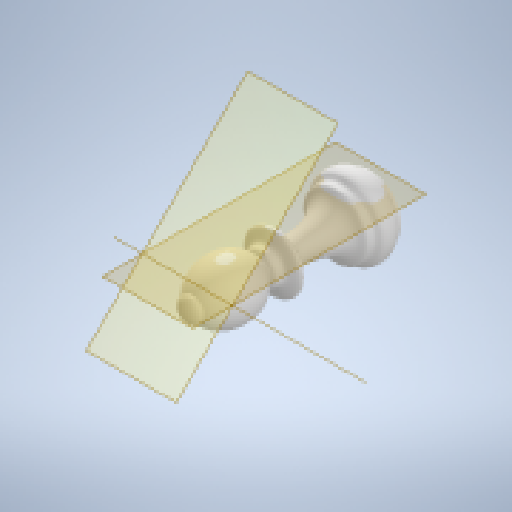
# Autodesk Inventor part: bishop-white
Saved by Autodesk Inventor 2024.1 (Build 281209000, 209)
## iProperties
Created: 2025-08-03
Part Number: bishop-white
Material: Generic
Document SubType Name: Modeling
Designer: iwheard
Density: 1 g/cm^3
Appearance: Default
Author: iwheard
Autodesk Inventor part; units mm, degrees
ref_plane "YZ Plane" through (0, 0, 0) normal (1, 0, 0) x (0, 1, 0)
ref_plane "XY Plane" through (0, 0, 0) normal (0, 0, 1) x (1, 0, 0)
sketch "Sketch1" plane through (0, 0, 0) normal (0, 0, 1) x (1, 0, 0)
  circle A0 centre (0, 25.5) radius 3
  circle A1 centre (0, 25.5) radius 5
  point P0 (0, 0)
  dimension "d0" = 10
  constraints: 2 centre point
  measures "d0" diameter of A1
extrude "Extrusion1" add sketch "Sketch1" along normal blind 3
sketch "Sketch3" plane through (0, 25.5, 3) normal (0, 0, 1) x (1, 0, 0)
  circle A0 centre (0, 0) radius 5 projected
  circle A1 centre (0, 0) radius 3 projected
  circle A2 centre (0, 0) radius 7.15
  point P0 (0, -25.5)
  dimension "d6" = 14.3
  constraints: 1 centre point
  measures "d6" diameter of A2
extrude "Extrusion2" add sketch "Sketch3" against normal blind 3 contours A2
sketch "Sketch2" plane through (0, 0, 0) normal (1, 0, 0) x (0, 1, 0)
  line L0 (30.5, 3) -> (20.5, 3) projected
  line L1 (30.5, 0) -> (20.5, 0) projected
  line L2 (30.5, 0) -> (30.5, 3) projected
  line L3 (28.5, 3) -> (28.5, 0) projected
  line L4 (32.65, 3) -> (18.35, 3) projected
  line L5 (32.65, 3) -> (32.65, 0) projected
  line L6 (28.3472, 21.8) -> (18.9472, 21.8)
  line L7 (19.95, 21.8) -> (32.25, 21.8)
  line L8 (32.65, 0.8) -> (33.5166, 1.2027) construction
  line L9 (33.5166, 1.2027) -> (34.0787, 2.2554) construction
  line L10 (34.0787, 2.2554) -> (34.4911, 4.0365) construction
  line L11 (34.4911, 4.0365) -> (34.2278, 5.2149) construction
  line L12 (34.2278, 5.2149) -> (33.7977, 5.9148) construction
  line L13 (33.7977, 5.9148) -> (33.0833, 6.0655) construction
  line L14 (33.0833, 6.0655) -> (32.65, 6.8872) construction
  line L15 (32.65, 6.8872) -> (33.4405, 8.43) construction
  line L16 (33.4405, 8.43) -> (29.4068, 8.43) construction
  line L17 (29.4068, 8.43) -> (27.9564, 17.9326) construction
  line L18 (32.25, 21.8) -> (32.25, 21.8) construction
  spline S0 degree 4 poles (32.65, 0.8) (33.5166, 1.2027) (34.0787, 2.2554) (34.4911, 4.0365) (34.2278, 5.2149) (33.7977, 5.9148) (33.0833, 6.0655) (32.65, 6.8872) (33.4405, 8.43) (29.4068, 8.43) (27.9564, 17.9326) (28.5, 20.0574) (31.3751, 21.1669) (32.1291, 21.5879) (32.2499, 21.7998) (32.25, 21.8) knots 1 1 1 1 1 2 3 4 5 6 7 8 9 10 10.505813 10.92418 11 11 11 11 11
  ellipse E0 centre (25.5, 41) end of major axis (22.7, 41) minor radius 1.4
  ellipse E1 centre (25.5, 33) end of major axis (25.5, 25) minor radius 6.5
  line L19 (32.25, 21.8) -> (32.4585, 22.7) construction
  line L20 (28.3607, 25.5724) -> (28.3108, 25.7867) construction
  spline S1 degree 4 poles (32.25, 21.8) (32.4585, 22.7) (29.8146, 23.2462) (29.2082, 23.4583) (29.4068, 25.3272) (28.3607, 25.5724) (28.3108, 25.7867) knots 1 1 1 1 1 1.620558 1.874487 2 2 2 2 2
  line L21 (29.4068, 25.3272) -> (28.3607, 25.5724) construction
  line L22 (32.4585, 22.7) -> (29.8146, 23.2462) construction
  line L23 (29.8146, 23.2462) -> (29.2082, 23.4583) construction
  line L24 (29.2082, 23.4583) -> (29.4068, 25.3272) construction
  line L25 (25.5, 42.4) -> (25.5, 3)
  line L26 (32.1291, 21.5879) -> (32.25, 21.8) construction
  line L27 (27.9564, 17.9326) -> (28.5, 20.0574) construction
  line L28 (28.5, 20.0574) -> (31.3751, 21.1669) construction
  line L29 (31.3751, 21.1669) -> (32.1291, 21.5879) construction
  point P0 (0, 0)
  point P1 (25.5, 0)
  point P2 (25.5, 3)
  point P3 (28.01, 40.3795)
  dimension "d127" = 2.8
  dimension "d128" = 1.4
  dimension "d129" = 6.5
  dimension "d130" = 8
  dimension "d89" = 12.3
  dimension "d131" = 8
  dimension "d132" = 33
  dimension "d133" = 11.2
  dimension "d134" = 6.75
  dimension "d135" = 0.8
  constraints: 6 end point, 3 midpoint, 3 vertical alignment, 2 coincident, 1 horizontal, 1 horizontal alignment, 1 point on line, 14 other
  measures "d89" distance of L7.end L7.start
  measures "d131" distance of point (25.5, 33) point (25.5, 41)
  measures "d132" distance from line of L1 point (25.5, 33)
  measures "d133" distance from line of point (25.5, 33) L6
  measures "d134" horizontal distance of point (32.25, 21.8) point (25.5, 33)
  measures "d135" distance from line of L8.start L1
revolve "Revolution1" add sketch "Sketch2" angle 360 about axis through (0, 25.5, 42.4) along (0, 0, -1) picked at (27.4668, 31.4146) picked at (26.1235, 40.0751) picked at (25.9921, 41.4318) contours L0 L25 L6 L7 S0 L5 L4 | L25 E1 S1 L7 L6 | L25 E0 E1 | L25 E1 E0 | E1 L25 E0
fillet "Fillet5" radius 0.6 1 edges at (0, 18.75, 21.8)
ref_plane "Work Plane6" through (0, 32, 33) normal (0, 1, 0) x (-1, 0, 0)
ref_plane "Work Plane9" through (0, 49.6777, 17.6777) normal (0, 0.7071068, 0.7071068) x (1, 0, 0)
ref_plane "Work Plane7" through (0, 32, 0) normal (0, 0.7071068, 0.7071068) x (1, 0, 0)
sketch "Sketch16" plane through (0, 49.6777, 17.6777) normal (0, 0.7071068, 0.7071068) x (1, 0, 0)
  line L0 (8, -30.0355) -> (0, -26.3614) construction
  line L1 (0, -26.3614) -> (-8, -30.0129) construction
  spline S0 degree 2 poles (8, -30.0355) (0, -26.3614) (-8, -30.0129) knots 1 1 1 2 2 2
  line L2 (8, -30.0355) -> (7.5, -28.6475)
  line L3 (-7.5, -28.6274) -> (-8, -30.0129)
  spline S1 degree 5 poles (7.5, -28.6475) (6.0737, -28.0663) (4.5989, -27.6042) (3.0818, -27.2819) (0.0019, -26.958) (-3.0789, -27.2731) (-4.5967, -27.5912) (-6.0725, -28.0496) (-7.5, -28.6274) knots 0 0 0 0 0 0 0.500029 0.500029 0.500029 1 1 1 1 1 1
  point P0 (0, -22.6274)
  point P1 (7.6736, -28.7905)
  point P2 (-7.681, -28.8125)
  point P3 (-4, -29.7611)
  point P4 (4, -29.7611)
  dimension "d137" = 8
  dimension "d138" = 8
  dimension "d141" = 6
  dimension "d142" = 7.5
  dimension "d143" = 7.5
  constraints: 4 end point, 1 vertical alignment, 6 other
  measures "d137" horizontal distance of L1.end point (0, -22.627)
  measures "d138" horizontal distance of L0.start point (0, -22.627)
  measures "d141" vertical distance of point (0, -22.627) L3.start
  measures "d142" horizontal distance of point (0, -22.627) L2.end
  measures "d143" horizontal distance of point (0, -22.627) L3.start
sketch "Sketch17" plane through (0, 0, 0) normal (1, 0, 0) x (0, 1, 0)
  line L0 (29.024, 39.7222) -> (29.1615, 34.9225) construction
  line L1 (29.1615, 34.9225) -> (26.7953, 31.6689) construction
  spline S0 degree 2 poles (29.024, 39.7222) (29.1615, 34.9225) (26.7953, 31.6689) knots 1 1 1 2 2 2
  point P0 (0, 0)
  constraints: 3 other
sweep "Sweep1" cut profiles "Sketch16" path "Sketch17"
sketch "Sketch15" plane through (0, 31.8, 41.7) normal (0, 0.7071068, -0.7071068) x (-1, 0, 0)
  line L0 (0, 3.0363) -> (2.0785, -0.5637)
  line L1 (2.0785, -0.5637) -> (-2.0785, -0.5637)
  line L2 (-2.0785, -0.5637) -> (0, 3.0363)
  ellipse E0 centre (0, -4.4548) end of major axis (-4.0302, -4.4548) minor radius 2.8498 projected
  ellipse E1 centre (0, -4.4548) end of major axis (-6.3, -4.4548) minor radius 4.4548 projected
  line L3 (2.0785, -0.5637) -> (0, -4.1637)
  line L4 (0, -4.1637) -> (-2.0785, -0.5637)
  line L5 (-2.0785, -0.5637) -> (2.0785, -0.5637)
  point P0 (0, -51.9723)
  point P1 (0, -14.238)
  point P2 (0, 0.6363)
  point P3 (0, -10.0471)
  point P4 (0, -1.7637)
  dimension "d118" = 2.4
  dimension "d51" = 6.0425
  dimension "d52" = 2.3149
  dimension "d53" = 2.4891
  dimension "d54" = 7.8751
  dimension "d55" = 5.9159
  dimension "d57" = 0.4873
  dimension "d58" = 0.2598
  dimension "d59" = 1.3529
  dimension "d60" = 2.0044
  dimension "d61" = 0.4355
  constraints: 72 end point, 18 parallel, 9 perpendicular, 6 point on line, 1 midpoint
sketch "Sketch12" plane through (-2.1873, 31.7347, 5.7495) normal (0, 0.6767574, 0.7362061) x (1, 0, 0)
  line L0 (7.0778, 4.6058) -> (7.2853, 4.1237)
  line L1 (7.2853, 4.1237) -> (7.7383, 3.6103)
  line L2 (7.7383, 3.6103) -> (8.2511, 3.1473)
  line L3 (8.2511, 3.1473) -> (8.8771, 3.0178)
  line L4 (8.8771, 3.0178) -> (9.2618, 2.9917)
  line L5 (9.2618, 2.9917) -> (9.5367, 3.0866)
  line L6 (9.5367, 3.0866) -> (10.2847, 4.0131)
  line L7 (10.2847, 4.0131) -> (10.6933, 4.6314)
  line L8 (10.6933, 4.6314) -> (10.7522, 4.8215)
  line L9 (10.7522, 4.8215) -> (10.6935, 4.9491)
  line L10 (10.6935, 4.9491) -> (10.1629, 5.066)
  line L11 (10.1629, 5.066) -> (8.9792, 5.0827)
  line L12 (8.9792, 5.0827) -> (7.1904, 5.0231)
  line L13 (7.1904, 5.0231) -> (7.0137, 4.8815)
  line L14 (7.0137, 4.8815) -> (7.0778, 4.6058)
  line L15 (-7.9123, 3.5374) -> (-6.7126, 2.2089)
  line L16 (-6.7126, 2.2089) -> (-6.4779, 2.096)
  line L17 (-6.4779, 2.096) -> (-6.283, 2.1812)
  line L18 (-6.283, 2.1812) -> (-5.9921, 2.5161)
  line L19 (-5.9921, 2.5161) -> (-5.7627, 3.7265)
  line L20 (-5.7627, 3.7265) -> (-5.6649, 4.5105)
  line L21 (-5.6649, 4.5105) -> (-5.802, 4.9132)
  line L22 (-5.802, 4.9132) -> (-6.3268, 5.0615)
  line L23 (-6.3268, 5.0615) -> (-7.392, 5.0827)
  line L24 (-7.392, 5.0827) -> (-8.4398, 5.0585)
  line L25 (-8.4398, 5.0585) -> (-8.8433, 4.8895)
  line L26 (-8.8433, 4.8895) -> (-8.6512, 4.4308)
  line L27 (-8.6512, 4.4308) -> (-7.9123, 3.5374)
  line L28 (0.8872, 3.9133) -> (0.9729, 2.8417)
  line L29 (0.9729, 2.8417) -> (1.3707, 2.3566)
  line L30 (1.3707, 2.3566) -> (1.8274, 2.0403)
  line L31 (1.8274, 2.0403) -> (2.3257, 2.1498)
  line L32 (2.3257, 2.1498) -> (2.6211, 2.2757)
  line L33 (2.6211, 2.2757) -> (2.7942, 2.4798)
  line L34 (2.7942, 2.4798) -> (3.0423, 3.7065)
  line L35 (3.0423, 3.7065) -> (3.1457, 4.5021)
  line L36 (3.1457, 4.5021) -> (3.0772, 4.9107)
  line L37 (3.0772, 4.9107) -> (2.7441, 5.0612)
  line L38 (2.7441, 5.0612) -> (2.0536, 5.0827)
  line L39 (2.0536, 5.0827) -> (1.3603, 5.0644)
  line L40 (1.3603, 5.0644) -> (1.0077, 4.9365)
  line L41 (1.0077, 4.9365) -> (0.8864, 4.5894)
  line L42 (0.8864, 4.5894) -> (0.8872, 3.9133)
  line L43 (-2.0027, 3.87) -> (-1.9541, 3.154)
  line L44 (-1.9541, 3.154) -> (-1.7644, 2.7594)
  line L45 (-1.7644, 2.7594) -> (-1.3586, 2.5882)
  line L46 (-1.3586, 2.5882) -> (-0.6615, 2.5421)
  line L47 (-0.6615, 2.5421) -> (0.3743, 2.5372)
  line L48 (0.3743, 2.5372) -> (0.6823, 2.6332)
  line L49 (0.6823, 2.6332) -> (0.8414, 2.878)
  line L50 (0.8414, 2.878) -> (0.8353, 3.9144)
  line L51 (0.8353, 3.9144) -> (0.7939, 4.5898)
  line L52 (0.7939, 4.5898) -> (0.6303, 4.9367)
  line L53 (0.6303, 4.9367) -> (0.2097, 5.0644)
  line L54 (0.2097, 5.0644) -> (-0.6026, 5.0827)
  line L55 (-0.6026, 5.0827) -> (-1.4144, 5.0637)
  line L56 (-1.4144, 5.0637) -> (-1.8308, 4.9311)
  line L57 (-1.8308, 4.9311) -> (-1.9832, 4.5711)
  line L58 (-1.9832, 4.5711) -> (-2.0027, 3.87)
  line L59 (-4.1807, 3.6112) -> (-4.1404, 2.7644)
  line L60 (-4.1404, 2.7644) -> (-4.0148, 2.3547)
  line L61 (-4.0148, 2.3547) -> (-3.7027, 2.2674)
  line L62 (-3.7027, 2.2674) -> (-3.1032, 2.3879)
  line L63 (-3.1032, 2.3879) -> (-2.4946, 2.5599)
  line L64 (-2.4946, 2.5599) -> (-2.1825, 2.7714)
  line L65 (-2.1825, 2.7714) -> (-2.0686, 3.161)
  line L66 (-2.0686, 3.161) -> (-2.0545, 3.8676)
  line L67 (-2.0545, 3.8676) -> (-2.0739, 4.5701)
  line L68 (-2.0739, 4.5701) -> (-2.1934, 4.9308)
  line L69 (-2.1934, 4.9308) -> (-2.515, 5.0637)
  line L70 (-2.515, 5.0637) -> (-3.1405, 5.0827)
  line L71 (-3.1405, 5.0827) -> (-3.7652, 5.0597)
  line L72 (-3.7652, 5.0597) -> (-4.0818, 4.8988)
  line L73 (-4.0818, 4.8988) -> (-4.1878, 4.4619)
  line L74 (-4.1878, 4.4619) -> (-4.1807, 3.6112)
  line L75 (-5.1318, 2.1686) -> (-4.4254, 1.9987)
  line L76 (-4.4254, 1.9987) -> (-4.2625, 2.0403)
  line L77 (-4.2625, 2.0403) -> (-4.2322, 3.5999)
  line L78 (-4.2322, 3.5999) -> (-4.3449, 4.8973)
  line L79 (-4.3449, 4.8973) -> (-4.5302, 5.0595)
  line L80 (-4.5302, 5.0595) -> (-4.8826, 5.0827)
  line L81 (-4.8826, 5.0827) -> (-5.2378, 5.0615)
  line L82 (-5.2378, 5.0615) -> (-5.4424, 4.9134)
  line L83 (-5.4424, 4.9134) -> (-5.7099, 3.7282)
  line L84 (-5.7099, 3.7282) -> (-5.824, 2.9419)
  line L85 (-5.824, 2.9419) -> (-5.8018, 2.5174)
  line L86 (-5.8018, 2.5174) -> (-5.5891, 2.3084)
  line L87 (-5.5891, 2.3084) -> (-5.1318, 2.1686)
  line L88 (3.6495, 2.0407) -> (4.1162, 1.9046)
  line L89 (4.1162, 1.9046) -> (4.4149, 2.0092)
  line L90 (4.4149, 2.0092) -> (4.6182, 2.4772)
  line L91 (4.6182, 2.4772) -> (4.7988, 3.4316)
  line L92 (4.7988, 3.4316) -> (4.9342, 4.3861)
  line L93 (4.9342, 4.3861) -> (4.915, 4.8762)
  line L94 (4.915, 4.8762) -> (4.6833, 5.0568)
  line L95 (4.6833, 5.0568) -> (4.1814, 5.0827)
  line L96 (4.1814, 5.0827) -> (3.6721, 5.0612)
  line L97 (3.6721, 5.0612) -> (3.3891, 4.9105)
  line L98 (3.3891, 4.9105) -> (3.2305, 4.5016)
  line L99 (3.2305, 4.5016) -> (3.0945, 3.7053)
  line L100 (3.0945, 3.7053) -> (2.9842, 2.9046)
  line L101 (2.9842, 2.9046) -> (3.0052, 2.4643)
  line L102 (3.0052, 2.4643) -> (3.2097, 2.2283)
  line L103 (3.2097, 2.2283) -> (3.6495, 2.0407)
  line L104 (9.8736, 2.3824) -> (10.0725, 2.0726)
  line L105 (10.0725, 2.0726) -> (10.3077, 1.9004)
  line L106 (10.3077, 1.9004) -> (11.4946, 1.7208)
  line L107 (11.4946, 1.7208) -> (12.2533, 1.6733)
  line L108 (12.2533, 1.6733) -> (12.6429, 1.8259)
  line L109 (12.6429, 1.8259) -> (12.7865, 2.33)
  line L110 (12.7865, 2.33) -> (12.8069, 3.3371)
  line L111 (12.8069, 3.3371) -> (12.7937, 4.3463)
  line L112 (12.7937, 4.3463) -> (12.701, 4.8645)
  line L113 (12.701, 4.8645) -> (12.4492, 5.0554)
  line L114 (12.4492, 5.0554) -> (11.959, 5.0827)
  line L115 (11.959, 5.0827) -> (11.4567, 5.0658)
  line L116 (11.4567, 5.0658) -> (11.1204, 4.9472)
  line L117 (11.1204, 4.9472) -> (10.338, 3.9987)
  line L118 (10.338, 3.9987) -> (9.7002, 2.9837)
  line L119 (9.7002, 2.9837) -> (9.7073, 2.7071)
  line L120 (9.7073, 2.7071) -> (9.8736, 2.3824)
  line L121 (4.9302, 1.5607) -> (5.2883, 1.3935)
  line L122 (5.2883, 1.3935) -> (5.7656, 1.4894)
  line L123 (5.7656, 1.4894) -> (6.0603, 1.5897)
  line L124 (6.0603, 1.5897) -> (6.2588, 1.7671)
  line L125 (6.2588, 1.7671) -> (6.7286, 2.8722)
  line L126 (6.7286, 2.8722) -> (7.1151, 4.0203)
  line L127 (7.1151, 4.0203) -> (7.0251, 4.5992)
  line L128 (7.0251, 4.5992) -> (6.768, 5.0224)
  line L129 (6.768, 5.0224) -> (5.9825, 5.0828)
  line L130 (5.9825, 5.0828) -> (5.4735, 5.0569)
  line L131 (5.4735, 5.0569) -> (5.1859, 4.8758)
  line L132 (5.1859, 4.8758) -> (5.0136, 4.3843)
  line L133 (5.0136, 4.3843) -> (4.8506, 3.4272)
  line L134 (4.8506, 3.4272) -> (4.6667, 1.9523)
  line L135 (4.6667, 1.9523) -> (4.7388, 1.7086)
  line L136 (4.7388, 1.7086) -> (4.9302, 1.5607)
  line L137 (-10.0996, 2.0946) -> (-9.1658, 1.7122)
  line L138 (-9.1658, 1.7122) -> (-7.9691, 1.6823)
  line L139 (-7.9691, 1.6823) -> (-6.8767, 1.7227)
  line L140 (-6.8767, 1.7227) -> (-6.6741, 1.8325)
  line L141 (-6.6741, 1.8325) -> (-6.7946, 2.1343)
  line L142 (-6.7946, 2.1343) -> (-7.9643, 3.5183)
  line L143 (-7.9643, 3.5183) -> (-9.2457, 4.8871)
  line L144 (-9.2457, 4.8871) -> (-9.6422, 5.0582)
  line L145 (-9.6422, 5.0582) -> (-10.1491, 5.0827)
  line L146 (-10.1491, 5.0827) -> (-10.6349, 5.0628)
  line L147 (-10.6349, 5.0628) -> (-10.8844, 4.9235)
  line L148 (-10.8844, 4.9235) -> (-10.9763, 4.5454)
  line L149 (-10.9763, 4.5454) -> (-10.9894, 3.8092)
  line L150 (-10.9894, 3.8092) -> (-10.9755, 3.0661)
  line L151 (-10.9755, 3.0661) -> (-10.8782, 2.6398)
  line L152 (-10.8782, 2.6398) -> (-10.614, 2.3696)
  line L153 (-10.614, 2.3696) -> (-10.0996, 2.0946)
  line L154 (7.0017, 1.241) -> (7.63, 0.9268)
  line L155 (7.63, 0.9268) -> (7.9057, 0.9992)
  line L156 (7.9057, 0.9992) -> (8.0999, 1.239)
  line L157 (8.0999, 1.239) -> (8.1581, 2.0966)
  line L158 (8.1581, 2.0966) -> (8.1291, 3.0002)
  line L159 (8.1291, 3.0002) -> (7.7126, 3.5622)
  line L160 (7.7126, 3.5622) -> (7.4273, 3.835)
  line L161 (7.4273, 3.835) -> (7.2344, 3.8511)
  line L162 (7.2344, 3.8511) -> (6.7731, 2.8435)
  line L163 (6.7731, 2.8435) -> (6.5187, 2.1301)
  line L164 (6.5187, 2.1301) -> (6.4577, 1.7254)
  line L165 (6.4577, 1.7254) -> (6.6116, 1.4791)
  line L166 (6.6116, 1.4791) -> (7.0017, 1.241)
  line L167 (8.7073, 1.062) -> (9.229, 1.0437)
  line L168 (9.229, 1.0437) -> (9.6868, 1.4053)
  line L169 (9.6868, 1.4053) -> (10.0394, 1.8435)
  line L170 (10.0394, 1.8435) -> (9.8261, 2.3611)
  line L171 (9.8261, 2.3611) -> (9.4772, 2.8348)
  line L172 (9.4772, 2.8348) -> (8.8815, 2.9651)
  line L173 (8.8815, 2.9651) -> (8.5129, 2.9925)
  line L174 (8.5129, 2.9925) -> (8.32, 2.9106)
  line L175 (8.32, 2.9106) -> (8.2098, 2.0909)
  line L176 (8.2098, 2.0909) -> (8.2457, 1.2518)
  line L177 (8.2457, 1.2518) -> (8.4, 1.124)
  line L178 (8.4, 1.124) -> (8.7073, 1.062)
  line L179 (-1.1975, 1.7234) -> (-0.675, 1.0352)
  line L180 (-0.675, 1.0352) -> (-0.4723, 0.9445)
  line L181 (-0.4723, 0.9445) -> (-0.2927, 1.0469)
  line L182 (-0.2927, 1.0469) -> (0.0688, 1.7112)
  line L183 (0.0688, 1.7112) -> (0.2778, 2.1497)
  line L184 (0.2778, 2.1497) -> (0.2719, 2.377)
  line L185 (0.2719, 2.377) -> (-0.0168, 2.4662)
  line L186 (-0.0168, 2.4662) -> (-0.6564, 2.4901)
  line L187 (-0.6564, 2.4901) -> (-1.2932, 2.4899)
  line L188 (-1.2932, 2.4899) -> (-1.5618, 2.41)
  line L189 (-1.5618, 2.41) -> (-1.513, 2.1784)
  line L190 (-1.513, 2.1784) -> (-1.1975, 1.7234)
  line L191 (-4.195, 1.1684) -> (-4.1205, 0.7334)
  line L192 (-4.1205, 0.7334) -> (-3.9979, 0.5322)
  line L193 (-3.9979, 0.5322) -> (-3.7448, 0.5165)
  line L194 (-3.7448, 0.5165) -> (-3.2787, 0.6377)
  line L195 (-3.2787, 0.6377) -> (-2.5542, 0.947)
  line L196 (-2.5542, 0.947) -> (-2.2838, 1.7234)
  line L197 (-2.2838, 1.7234) -> (-2.1873, 2.2134)
  line L198 (-2.1873, 2.2134) -> (-2.2423, 2.44)
  line L199 (-2.2423, 2.44) -> (-2.5269, 2.4601)
  line L200 (-2.5269, 2.4601) -> (-3.1198, 2.3307)
  line L201 (-3.1198, 2.3307) -> (-4.2248, 2.0047)
  line L202 (-4.2248, 2.0047) -> (-4.195, 1.1684)
  line L203 (0.319, 0.4663) -> (0.6686, 0.2086)
  line L204 (0.6686, 0.2086) -> (0.8924, 0.1637)
  line L205 (0.8924, 0.1637) -> (1.087, 0.3684)
  line L206 (1.087, 0.3684) -> (1.3488, 0.8597)
  line L207 (1.3488, 0.8597) -> (1.6779, 1.8428)
  line L208 (1.6779, 1.8428) -> (1.593, 2.0742)
  line L209 (1.593, 2.0742) -> (1.3408, 2.314)
  line L210 (1.3408, 2.314) -> (0.9255, 2.6376)
  line L211 (0.9255, 2.6376) -> (0.7075, 2.5879)
  line L212 (0.7075, 2.5879) -> (0.4957, 2.3936)
  line L213 (0.4957, 2.3936) -> (0.1242, 1.7056)
  line L214 (0.1242, 1.7056) -> (-0.15, 0.973)
  line L215 (-0.15, 0.973) -> (-0.0175, 0.7495)
  line L216 (-0.0175, 0.7495) -> (0.319, 0.4663)
  line L217 (2.5187, 0.9763) -> (2.9216, 0.5547)
  line L218 (2.9216, 0.5547) -> (3.1879, 0.4137)
  line L219 (3.1879, 0.4137) -> (3.4364, 0.5525)
  line L220 (3.4364, 0.5525) -> (3.7858, 0.9708)
  line L221 (3.7858, 0.9708) -> (4.1127, 1.4052)
  line L222 (4.1127, 1.4052) -> (4.2037, 1.6573)
  line L223 (4.2037, 1.6573) -> (4.0425, 1.823)
  line L224 (4.0425, 1.823) -> (3.6129, 1.9991)
  line L225 (3.6129, 1.9991) -> (2.8855, 2.2254)
  line L226 (2.8855, 2.2254) -> (2.3473, 2.1025)
  line L227 (2.3473, 2.1025) -> (2.0633, 1.8728)
  line L228 (2.0633, 1.8728) -> (1.9865, 1.679)
  line L229 (1.9865, 1.679) -> (2.5187, 0.9763)
  line L230 (-6.6273, 0.9505) -> (-6.5332, 0.2753)
  line L231 (-6.5332, 0.2753) -> (-6.2216, -0.0684)
  line L232 (-6.2216, -0.0684) -> (-5.6991, -0.3658)
  line L233 (-5.6991, -0.3658) -> (-4.8336, 0.0157)
  line L234 (-4.8336, 0.0157) -> (-4.242, 0.4515)
  line L235 (-4.242, 0.4515) -> (-4.2462, 1.1599)
  line L236 (-4.2462, 1.1599) -> (-4.437, 1.8453)
  line L237 (-4.437, 1.8453) -> (-5.1517, 2.1202)
  line L238 (-5.1517, 2.1202) -> (-5.8919, 2.2767)
  line L239 (-5.8919, 2.2767) -> (-6.2614, 2.1336)
  line L240 (-6.2614, 2.1336) -> (-6.627, 1.8108)
  line L241 (-6.627, 1.8108) -> (-6.6273, 0.9505)
  line L242 (-6.6273, 0.9505) -> (-6.6273, 0.9505)
  line L243 (-1.9958, 0.4442) -> (-1.5615, 0.1379)
  line L244 (-1.5615, 0.1379) -> (-1.1159, 0.4715)
  line L245 (-1.1159, 0.4715) -> (-0.8663, 0.7386)
  line L246 (-0.8663, 0.7386) -> (-0.7977, 0.9571)
  line L247 (-0.7977, 0.9571) -> (-1.2554, 1.7148)
  line L248 (-1.2554, 1.7148) -> (-1.7069, 2.2125)
  line L249 (-1.7069, 2.2125) -> (-1.9588, 2.3798)
  line L250 (-1.9588, 2.3798) -> (-2.1026, 2.2179)
  line L251 (-2.1026, 2.2179) -> (-2.2295, 1.7281)
  line L252 (-2.2295, 1.7281) -> (-2.3493, 0.9143)
  line L253 (-2.3493, 0.9143) -> (-1.9958, 0.4442)
  line L254 (-8.5605, 0.7102) -> (-7.9464, -0.0451)
  line L255 (-7.9464, -0.0451) -> (-7.6823, -0.0821)
  line L256 (-7.6823, -0.0821) -> (-7.2878, 0.0218)
  line L257 (-7.2878, 0.0218) -> (-6.7123, 0.2899)
  line L258 (-6.7123, 0.2899) -> (-6.6787, 0.9424)
  line L259 (-6.6787, 0.9424) -> (-6.7305, 1.3563)
  line L260 (-6.7305, 1.3563) -> (-6.8803, 1.566)
  line L261 (-6.8803, 1.566) -> (-7.9513, 1.6308)
  line L262 (-7.9513, 1.6308) -> (-8.6448, 1.6006)
  line L263 (-8.6448, 1.6006) -> (-8.9394, 1.4946)
  line L264 (-8.9394, 1.4946) -> (-8.8923, 1.2266)
  line L265 (-8.8923, 1.2266) -> (-8.5605, 0.7102)
  line L266 (9.5166, 0.3752) -> (9.6778, 0.049)
  line L267 (9.6778, 0.049) -> (9.9152, -0.0926)
  line L268 (9.9152, -0.0926) -> (11.2805, 0.0602)
  line L269 (11.2805, 0.0602) -> (12.6162, 0.3608)
  line L270 (12.6162, 0.3608) -> (12.7831, 0.5703)
  line L271 (12.7831, 0.5703) -> (12.807, 0.9279)
  line L272 (12.807, 0.9279) -> (12.7864, 1.2835)
  line L273 (12.7864, 1.2835) -> (12.6425, 1.4792)
  line L274 (12.6425, 1.4792) -> (11.4914, 1.669)
  line L275 (11.4914, 1.669) -> (10.2842, 1.7291)
  line L276 (10.2842, 1.7291) -> (10.0072, 1.6167)
  line L277 (10.0072, 1.6167) -> (9.7274, 1.3724)
  line L278 (9.7274, 1.3724) -> (9.3649, 0.9281)
  line L279 (9.3649, 0.9281) -> (9.5166, 0.3752)
  line L280 (1.3913, -0.4022) -> (1.8487, -0.6499)
  line L281 (1.8487, -0.6499) -> (2.4597, -0.593)
  line L282 (2.4597, -0.593) -> (3.0216, -0.4573)
  line L283 (3.0216, -0.4573) -> (3.1352, -0.1535)
  line L284 (3.1352, -0.1535) -> (3.0845, 0.23)
  line L285 (3.0845, 0.23) -> (2.4959, 0.9243)
  line L286 (2.4959, 0.9243) -> (2.097, 1.3422)
  line L287 (2.097, 1.3422) -> (1.8481, 1.4698)
  line L288 (1.8481, 1.4698) -> (1.6448, 1.2966)
  line L289 (1.6448, 1.2966) -> (1.3828, 0.812)
  line L290 (1.3828, 0.812) -> (1.0664, -0.0265)
  line L291 (1.0664, -0.0265) -> (1.1483, -0.2153)
  line L292 (1.1483, -0.2153) -> (1.3913, -0.4022)
  line L293 (5.3624, 0.5254) -> (5.5243, -0.1888)
  line L294 (5.5243, -0.1888) -> (6.2364, -0.5262)
  line L295 (6.2364, -0.5262) -> (6.9598, -0.7576)
  line L296 (6.9598, -0.7576) -> (7.2022, -0.7304)
  line L297 (7.2022, -0.7304) -> (7.3626, -0.5765)
  line L298 (7.3626, -0.5765) -> (7.5125, 0.0792)
  line L299 (7.5125, 0.0792) -> (7.5557, 0.7738)
  line L300 (7.5557, 0.7738) -> (6.9699, 1.1993)
  line L301 (6.9699, 1.1993) -> (6.3038, 1.5151)
  line L302 (6.3038, 1.5151) -> (5.7857, 1.4412)
  line L303 (5.7857, 1.4412) -> (5.3626, 1.2226)
  line L304 (5.3626, 1.2226) -> (5.3624, 0.5254)
  line L305 (3.2595, -0.5938) -> (4.0875, -0.7338)
  line L306 (4.0875, -0.7338) -> (4.7497, -0.7393)
  line L307 (4.7497, -0.7393) -> (5.0922, -0.5185)
  line L308 (5.0922, -0.5185) -> (5.3364, -0.1945)
  line L309 (5.3364, -0.1945) -> (5.3106, 0.5231)
  line L310 (5.3106, 0.5231) -> (5.206, 1.235)
  line L311 (5.206, 1.235) -> (4.8994, 1.5188)
  line L312 (4.8994, 1.5188) -> (4.6179, 1.6134)
  line L313 (4.6179, 1.6134) -> (4.4124, 1.5846)
  line L314 (4.4124, 1.5846) -> (3.8274, 0.9398)
  line L315 (3.8274, 0.9398) -> (3.2964, 0.23)
  line L316 (3.2964, 0.23) -> (3.1867, -0.1601)
  line L317 (3.1867, -0.1601) -> (3.1662, -0.467)
  line L318 (3.1662, -0.467) -> (3.2595, -0.5938)
  line L319 (-9.8289, -0.9114) -> (-8.7715, -0.9751)
  line L320 (-8.7715, -0.9751) -> (-8.5448, -0.866)
  line L321 (-8.5448, -0.866) -> (-8.3325, -0.6274)
  line L322 (-8.3325, -0.6274) -> (-8.148, -0.3726)
  line L323 (-8.148, -0.3726) -> (-8.1159, -0.1496)
  line L324 (-8.1159, -0.1496) -> (-8.6149, 0.698)
  line L325 (-8.6149, 0.698) -> (-9.2656, 1.548)
  line L326 (-9.2656, 1.548) -> (-10.1113, 2.0426)
  line L327 (-10.1113, 2.0426) -> (-10.6189, 2.2688)
  line L328 (-10.6189, 2.2688) -> (-10.8797, 2.2199)
  line L329 (-10.8797, 2.2199) -> (-10.9757, 1.7841)
  line L330 (-10.9757, 1.7841) -> (-10.9894, 0.8493)
  line L331 (-10.9894, 0.8493) -> (-10.9713, -0.0942)
  line L332 (-10.9713, -0.0942) -> (-10.8444, -0.5922)
  line L333 (-10.8444, -0.5922) -> (-10.4998, -0.8096)
  line L334 (-10.4998, -0.8096) -> (-9.8289, -0.9114)
  line L335 (8.2447, -1.1136) -> (8.7357, -1.3578)
  line L336 (8.7357, -1.3578) -> (9.0302, -1.4084)
  line L337 (9.0302, -1.4084) -> (9.2246, -1.2525)
  line L338 (9.2246, -1.2525) -> (9.4153, -0.8771)
  line L339 (9.4153, -0.8771) -> (9.643, -0.234)
  line L340 (9.643, -0.234) -> (9.4699, 0.3524)
  line L341 (9.4699, 0.3524) -> (9.1927, 0.8676)
  line L342 (9.1927, 0.8676) -> (8.6918, 1.0119)
  line L343 (8.6918, 1.0119) -> (8.1934, 1.0667)
  line L344 (8.1934, 1.0667) -> (7.9333, 0.9553)
  line L345 (7.9333, 0.9553) -> (7.7219, 0.7411)
  line L346 (7.7219, 0.7411) -> (7.5646, 0.0757)
  line L347 (7.5646, 0.0757) -> (7.4918, -0.3594)
  line L348 (7.4918, -0.3594) -> (7.5384, -0.6284)
  line L349 (7.5384, -0.6284) -> (8.2447, -1.1136)
  line L350 (-3.269, -0.6766) -> (-2.5401, -1.5703)
  line L351 (-2.5401, -1.5703) -> (-2.3211, -1.6435)
  line L352 (-2.3211, -1.6435) -> (-2.046, -1.5805)
  line L353 (-2.046, -1.5805) -> (-1.6478, -1.3713)
  line L354 (-1.6478, -1.3713) -> (-1.5901, -0.7296)
  line L355 (-1.5901, -0.7296) -> (-1.6439, -0.0529)
  line L356 (-1.6439, -0.0529) -> (-2.0264, 0.4018)
  line L357 (-2.0264, 0.4018) -> (-2.5074, 0.7388)
  line L358 (-2.5074, 0.7388) -> (-3.2503, 0.5919)
  line L359 (-3.2503, 0.5919) -> (-3.6931, 0.4441)
  line L360 (-3.6931, 0.4441) -> (-3.8426, 0.2627)
  line L361 (-3.8426, 0.2627) -> (-3.7006, -0.0712)
  line L362 (-3.7006, -0.0712) -> (-3.269, -0.6766)
  line L363 (-1.0434, -1.4148) -> (-0.5343, -1.3024)
  line L364 (-0.5343, -1.3024) -> (0.1704, -0.7431)
  line L365 (0.1704, -0.7431) -> (0.5811, -0.3391)
  line L366 (0.5811, -0.3391) -> (0.7306, -0.083)
  line L367 (0.7306, -0.083) -> (0.6301, 0.1344)
  line L368 (0.6301, 0.1344) -> (0.2911, 0.4223)
  line L369 (0.2911, 0.4223) -> (-0.2585, 0.8407)
  line L370 (-0.2585, 0.8407) -> (-0.469, 0.8927)
  line L371 (-0.469, 0.8927) -> (-0.6609, 0.8286)
  line L372 (-0.6609, 0.8286) -> (-1.0801, 0.434)
  line L373 (-1.0801, 0.434) -> (-1.4802, -0.0488)
  line L374 (-1.4802, -0.0488) -> (-1.5382, -0.7304)
  line L375 (-1.5382, -0.7304) -> (-1.4626, -1.3577)
  line L376 (-1.4626, -1.3577) -> (-1.0434, -1.4148)
  line L377 (10.6927, -1.6839) -> (12.0541, -1.8125)
  line L378 (12.0541, -1.8125) -> (12.5063, -1.758)
  line L379 (12.5063, -1.758) -> (12.6801, -1.6937)
  line L380 (12.6801, -1.6937) -> (12.7694, -1.5625)
  line L381 (12.7694, -1.5625) -> (12.8069, -0.7046)
  line L382 (12.8069, -0.7046) -> (12.7831, -0.1488)
  line L383 (12.7831, -0.1488) -> (12.6163, 0.1107)
  line L384 (12.6163, 0.1107) -> (12.1634, 0.1406)
  line L385 (12.1634, 0.1406) -> (11.2815, 0.0078)
  line L386 (11.2815, 0.0078) -> (9.9107, -0.296)
  line L387 (9.9107, -0.296) -> (9.6583, -0.5135)
  line L388 (9.6583, -0.5135) -> (9.4679, -0.8866)
  line L389 (9.4679, -0.8866) -> (9.3249, -1.2581)
  line L390 (9.3249, -1.2581) -> (9.4049, -1.465)
  line L391 (9.4049, -1.465) -> (10.6927, -1.6839)
  line L392 (-4.8865, -1.3487) -> (-4.2822, -2.1641)
  line L393 (-4.2822, -2.1641) -> (-4.0193, -2.2528)
  line L394 (-4.0193, -2.2528) -> (-3.625, -2.2404)
  line L395 (-3.625, -2.2404) -> (-3.0163, -2.1714)
  line L396 (-3.0163, -2.1714) -> (-2.7518, -1.9696)
  line L397 (-2.7518, -1.9696) -> (-2.6441, -1.8238)
  line L398 (-2.6441, -1.8238) -> (-2.6675, -1.6423)
  line L399 (-2.6675, -1.6423) -> (-3.3204, -0.6942)
  line L400 (-3.3204, -0.6942) -> (-3.789, -0.0887)
  line L401 (-3.789, -0.0887) -> (-4.099, 0.183)
  line L402 (-4.099, 0.183) -> (-4.3889, 0.1839)
  line L403 (-4.3889, 0.1839) -> (-4.7971, -0.0233)
  line L404 (-4.7971, -0.0233) -> (-5.1837, -0.2616)
  line L405 (-5.1837, -0.2616) -> (-5.3219, -0.4791)
  line L406 (-5.3219, -0.4791) -> (-5.22, -0.8001)
  line L407 (-5.22, -0.8001) -> (-4.8865, -1.3487)
  line L408 (-8.3905, -1.5272) -> (-8.0877, -1.9226)
  line L409 (-8.0877, -1.9226) -> (-7.3827, -1.9719)
  line L410 (-7.3827, -1.9719) -> (-6.6638, -1.8661)
  line L411 (-6.6638, -1.8661) -> (-6.263, -1.1766)
  line L412 (-6.263, -1.1766) -> (-6.0015, -0.4526)
  line L413 (-6.0015, -0.4526) -> (-6.0651, -0.2822)
  line L414 (-6.0651, -0.2822) -> (-6.2577, -0.1057)
  line L415 (-6.2577, -0.1057) -> (-6.6417, 0.1169)
  line L416 (-6.6417, 0.1169) -> (-7.2747, -0.0284)
  line L417 (-7.2747, -0.0284) -> (-7.9073, -0.2616)
  line L418 (-7.9073, -0.2616) -> (-8.2878, -0.6545)
  line L419 (-8.2878, -0.6545) -> (-8.5545, -1.0783)
  line L420 (-8.5545, -1.0783) -> (-8.3905, -1.5272)
  line L421 (5.0506, -1.8975) -> (5.2494, -2.8598)
  line L422 (5.2494, -2.8598) -> (5.3797, -3.0892)
  line L423 (5.3797, -3.0892) -> (5.5342, -3.1679)
  line L424 (5.5342, -3.1679) -> (5.856, -3.0612)
  line L425 (5.856, -3.0612) -> (6.2121, -2.8109)
  line L426 (6.2121, -2.8109) -> (6.6066, -1.884)
  line L427 (6.6066, -1.884) -> (6.8259, -1.2787)
  line L428 (6.8259, -1.2787) -> (6.8577, -0.9402)
  line L429 (6.8577, -0.9402) -> (6.665, -0.7457)
  line L430 (6.665, -0.7457) -> (6.2108, -0.5722)
  line L431 (6.2108, -0.5722) -> (5.4781, -0.3662)
  line L432 (5.4781, -0.3662) -> (5.1274, -0.5566)
  line L433 (5.1274, -0.5566) -> (4.9648, -0.7218)
  line L434 (4.9648, -0.7218) -> (4.9026, -0.9166)
  line L435 (4.9026, -0.9166) -> (5.0506, -1.8975)
  line L436 (0.0881, -1.9045) -> (0.6712, -2.3329)
  line L437 (0.6712, -2.3329) -> (1.1262, -2.3149)
  line L438 (1.1262, -2.3149) -> (1.52, -2.1415)
  line L439 (1.52, -2.1415) -> (1.6743, -1.4813)
  line L440 (1.6743, -1.4813) -> (1.7214, -0.796)
  line L441 (1.7214, -0.796) -> (1.3634, -0.4459)
  line L442 (1.3634, -0.4459) -> (1.106, -0.2856)
  line L443 (1.106, -0.2856) -> (0.9002, -0.2666)
  line L444 (0.9002, -0.2666) -> (0.2108, -0.7768)
  line L445 (0.2108, -0.7768) -> (-0.2001, -1.146)
  line L446 (-0.2001, -1.146) -> (-0.3498, -1.3865)
  line L447 (-0.3498, -1.3865) -> (-0.2499, -1.6041)
  line L448 (-0.2499, -1.6041) -> (0.0881, -1.9045)
  line L449 (1.9705, -2.5646) -> (2.5287, -2.9313)
  line L450 (2.5287, -2.9313) -> (2.7391, -2.9405)
  line L451 (2.7391, -2.9405) -> (3.0217, -2.7843)
  line L452 (3.0217, -2.7843) -> (3.2807, -2.5066)
  line L453 (3.2807, -2.5066) -> (3.3259, -1.6642)
  line L454 (3.3259, -1.6642) -> (3.3204, -0.8327)
  line L455 (3.3204, -0.8327) -> (3.2238, -0.6314)
  line L456 (3.2238, -0.6314) -> (3.0466, -0.5606)
  line L457 (3.0466, -0.5606) -> (2.476, -0.6428)
  line L458 (2.476, -0.6428) -> (1.905, -0.8298)
  line L459 (1.905, -0.8298) -> (1.7251, -1.4925)
  line L460 (1.7251, -1.4925) -> (1.6698, -2.183)
  line L461 (1.6698, -2.183) -> (1.9705, -2.5646)
  line L462 (4.2862, -2.7782) -> (4.8137, -2.868)
  line L463 (4.8137, -2.868) -> (5.0636, -2.806)
  line L464 (5.0636, -2.806) -> (5.1026, -2.5094)
  line L465 (5.1026, -2.5094) -> (4.9974, -1.8953)
  line L466 (4.9974, -1.8953) -> (4.7288, -0.9563)
  line L467 (4.7288, -0.9563) -> (4.4978, -0.827)
  line L468 (4.4978, -0.827) -> (4.0889, -0.7858)
  line L469 (4.0889, -0.7858) -> (3.6831, -0.7758)
  line L470 (3.6831, -0.7758) -> (3.4738, -0.8644)
  line L471 (3.4738, -0.8644) -> (3.3777, -1.6687)
  line L472 (3.3777, -1.6687) -> (3.3866, -2.2065)
  line L473 (3.3866, -2.2065) -> (3.4842, -2.5013)
  line L474 (3.4842, -2.5013) -> (3.7557, -2.6572)
  line L475 (3.7557, -2.6572) -> (4.2862, -2.7782)
  line L476 (-6.4089, -2.3236) -> (-6.1803, -2.6239)
  line L477 (-6.1803, -2.6239) -> (-5.519, -2.718)
  line L478 (-5.519, -2.718) -> (-4.8492, -2.741)
  line L479 (-4.8492, -2.741) -> (-4.5615, -2.5443)
  line L480 (-4.5615, -2.5443) -> (-4.4413, -2.3947)
  line L481 (-4.4413, -2.3947) -> (-4.4402, -2.2223)
  line L482 (-4.4402, -2.2223) -> (-4.9353, -1.3686)
  line L483 (-4.9353, -1.3686) -> (-5.4792, -0.5429)
  line L484 (-5.4792, -0.5429) -> (-5.7001, -0.4176)
  line L485 (-5.7001, -0.4176) -> (-5.8898, -0.5089)
  line L486 (-5.8898, -0.5089) -> (-6.2162, -1.199)
  line L487 (-6.2162, -1.199) -> (-6.5022, -1.9319)
  line L488 (-6.5022, -1.9319) -> (-6.4089, -2.3236)
  line L489 (7.0181, -3.1437) -> (7.4662, -3.2559)
  line L490 (7.4662, -3.2559) -> (7.7605, -3.2257)
  line L491 (7.7605, -3.2257) -> (8.4099, -2.4956)
  line L492 (8.4099, -2.4956) -> (8.7651, -1.9749)
  line L493 (8.7651, -1.9749) -> (8.8634, -1.6619)
  line L494 (8.8634, -1.6619) -> (8.6865, -1.4312)
  line L495 (8.6865, -1.4312) -> (8.2163, -1.1572)
  line L496 (8.2163, -1.1572) -> (7.4694, -0.7723)
  line L497 (7.4694, -0.7723) -> (7.2237, -0.7776)
  line L498 (7.2237, -0.7776) -> (7.0317, -0.969)
  line L499 (7.0317, -0.969) -> (6.6608, -1.8871)
  line L500 (6.6608, -1.8871) -> (6.441, -2.4914)
  line L501 (6.441, -2.4914) -> (6.405, -2.8237)
  line L502 (6.405, -2.8237) -> (6.5862, -3.0019)
  line L503 (6.5862, -3.0019) -> (7.0181, -3.1437)
  line L504 (-9.8221, -3.7074) -> (-9.1436, -3.6665)
  line L505 (-9.1436, -3.6665) -> (-8.7721, -3.5619)
  line L506 (-8.7721, -3.5619) -> (-8.5766, -3.3117)
  line L507 (-8.5766, -3.3117) -> (-8.4264, -2.8341)
  line L508 (-8.4264, -2.8341) -> (-8.2563, -2.0553)
  line L509 (-8.2563, -2.0553) -> (-8.4359, -1.5523)
  line L510 (-8.4359, -1.5523) -> (-8.5915, -1.286)
  line L511 (-8.5915, -1.286) -> (-8.7888, -1.1359)
  line L512 (-8.7888, -1.1359) -> (-9.8316, -0.9633)
  line L513 (-9.8316, -0.9633) -> (-10.501, -0.9099)
  line L514 (-10.501, -0.9099) -> (-10.8447, -1.0307)
  line L515 (-10.8447, -1.0307) -> (-10.9713, -1.4504)
  line L516 (-10.9713, -1.4504) -> (-10.9894, -2.2937)
  line L517 (-10.9894, -2.2937) -> (-10.9712, -3.1383)
  line L518 (-10.9712, -3.1383) -> (-10.8435, -3.5671)
  line L519 (-10.8435, -3.5671) -> (-10.4969, -3.7127)
  line L520 (-10.4969, -3.7127) -> (-9.8221, -3.7074)
  line L521 (9.6212, -2.6112) -> (9.9509, -3.1628)
  line L522 (9.9509, -3.1628) -> (10.236, -3.3608)
  line L523 (10.236, -3.3608) -> (10.6037, -3.2162)
  line L524 (10.6037, -3.2162) -> (11.1808, -2.74)
  line L525 (11.1808, -2.74) -> (11.7156, -2.2455)
  line L526 (11.7156, -2.2455) -> (11.8383, -1.9756)
  line L527 (11.8383, -1.9756) -> (11.4989, -1.8357)
  line L528 (11.4989, -1.8357) -> (10.6473, -1.7313)
  line L529 (10.6473, -1.7313) -> (9.7583, -1.6909)
  line L530 (9.7583, -1.6909) -> (9.3551, -1.7691)
  line L531 (9.3551, -1.7691) -> (9.3415, -2.0484)
  line L532 (9.3415, -2.0484) -> (9.6212, -2.6112)
  line L533 (-1.1041, -2.5543) -> (-0.7031, -3.4576)
  line L534 (-0.7031, -3.4576) -> (-0.506, -3.5317)
  line L535 (-0.506, -3.5317) -> (-0.1981, -3.4682)
  line L536 (-0.1981, -3.4682) -> (0.2796, -3.2918)
  line L537 (0.2796, -3.2918) -> (0.4896, -2.8866)
  line L538 (0.4896, -2.8866) -> (0.558, -2.4354)
  line L539 (0.558, -2.4354) -> (0.045, -1.9361)
  line L540 (0.045, -1.9361) -> (-0.5463, -1.4968)
  line L541 (-0.5463, -1.4968) -> (-1.0263, -1.4655)
  line L542 (-1.0263, -1.4655) -> (-1.2871, -1.5031)
  line L543 (-1.2871, -1.5031) -> (-1.3821, -1.6291)
  line L544 (-1.3821, -1.6291) -> (-1.1041, -2.5543)
  line L545 (-7.6168, -3.6137) -> (-6.7523, -3.4892)
  line L546 (-6.7523, -3.4892) -> (-6.4761, -3.1077)
  line L547 (-6.4761, -3.1077) -> (-6.3397, -2.6947)
  line L548 (-6.3397, -2.6947) -> (-6.4541, -2.3494)
  line L549 (-6.4541, -2.3494) -> (-6.687, -2.0581)
  line L550 (-6.687, -2.0581) -> (-7.3804, -2.0237)
  line L551 (-7.3804, -2.0237) -> (-7.8292, -2.0414)
  line L552 (-7.8292, -2.0414) -> (-8.0827, -2.1337)
  line L553 (-8.0827, -2.1337) -> (-8.3779, -2.8533)
  line L554 (-8.3779, -2.8533) -> (-8.4794, -3.3389)
  line L555 (-8.4794, -3.3389) -> (-8.4339, -3.58)
  line L556 (-8.4339, -3.58) -> (-8.1702, -3.6478)
  line L557 (-8.1702, -3.6478) -> (-7.6168, -3.6137)
  line L558 (7.9052, -3.5671) -> (8.0584, -3.7567)
  line L559 (8.0584, -3.7567) -> (8.5982, -4.0421)
  line L560 (8.5982, -4.0421) -> (9.1829, -4.2597)
  line L561 (9.1829, -4.2597) -> (9.6503, -3.9747)
  line L562 (9.6503, -3.9747) -> (9.9011, -3.7466)
  line L563 (9.9011, -3.7466) -> (9.9775, -3.5322)
  line L564 (9.9775, -3.5322) -> (9.5817, -2.6472)
  line L565 (9.5817, -2.6472) -> (9.2734, -2.1062)
  line L566 (9.2734, -2.1062) -> (9.0518, -1.9148)
  line L567 (9.0518, -1.9148) -> (8.81, -2.0631)
  line L568 (8.81, -2.0631) -> (8.4409, -2.5409)
  line L569 (8.4409, -2.5409) -> (7.9057, -3.3085)
  line L570 (7.9057, -3.3085) -> (7.9052, -3.5671)
  line L571 (0.7591, -3.7719) -> (0.9908, -4.0083)
  line L572 (0.9908, -4.0083) -> (1.1674, -4.0649)
  line L573 (1.1674, -4.0649) -> (1.7133, -3.5593)
  line L574 (1.7133, -3.5593) -> (2.1668, -2.9599)
  line L575 (2.1668, -2.9599) -> (2.1241, -2.7938)
  line L576 (2.1241, -2.7938) -> (1.9286, -2.5965)
  line L577 (1.9286, -2.5965) -> (1.5649, -2.3245)
  line L578 (1.5649, -2.3245) -> (1.14, -2.365)
  line L579 (1.14, -2.365) -> (0.7386, -2.5015)
  line L580 (0.7386, -2.5015) -> (0.5393, -2.9017)
  line L581 (0.5393, -2.9017) -> (0.4426, -3.3436)
  line L582 (0.4426, -3.3436) -> (0.7591, -3.7719)
  line L583 (-2.8282, -3.0588) -> (-2.6785, -3.8206)
  line L584 (-2.6785, -3.8206) -> (-2.1797, -4.1658)
  line L585 (-2.1797, -4.1658) -> (-1.6558, -4.3922)
  line L586 (-1.6558, -4.3922) -> (-1.3307, -4.323)
  line L587 (-1.3307, -4.323) -> (-1.0581, -4.1837)
  line L588 (-1.0581, -4.1837) -> (-0.9017, -3.9203)
  line L589 (-0.9017, -3.9203) -> (-0.8305, -3.5381)
  line L590 (-0.8305, -3.5381) -> (-1.1545, -2.5675)
  line L591 (-1.1545, -2.5675) -> (-1.573, -1.6423)
  line L592 (-1.573, -1.6423) -> (-1.7561, -1.5661)
  line L593 (-1.7561, -1.5661) -> (-2.0315, -1.6303)
  line L594 (-2.0315, -1.6303) -> (-2.4651, -1.7815)
  line L595 (-2.4651, -1.7815) -> (-2.7083, -1.999)
  line L596 (-2.7083, -1.999) -> (-2.8819, -2.3029)
  line L597 (-2.8819, -2.3029) -> (-2.8282, -3.0588)
  line L598 (-6.3035, -4.0622) -> (-5.9636, -4.5121)
  line L599 (-5.9636, -4.5121) -> (-5.4079, -4.6147)
  line L600 (-5.4079, -4.6147) -> (-5.0657, -4.6262)
  line L601 (-5.0657, -4.6262) -> (-4.8893, -4.5393)
  line L602 (-4.8893, -4.5393) -> (-4.8089, -3.7439)
  line L603 (-4.8089, -3.7439) -> (-4.8931, -2.9354)
  line L604 (-4.8931, -2.9354) -> (-5.1078, -2.8178)
  line L605 (-5.1078, -2.8178) -> (-5.5272, -2.7693)
  line L606 (-5.5272, -2.7693) -> (-6.1843, -2.7704)
  line L607 (-6.1843, -2.7704) -> (-6.4302, -3.1324)
  line L608 (-6.4302, -3.1324) -> (-6.5473, -3.5652)
  line L609 (-6.5473, -3.5652) -> (-6.3035, -4.0622)
  line L610 (-4.5225, -4.8817) -> (-4.3709, -4.9916)
  line L611 (-4.3709, -4.9916) -> (-4.2174, -4.9877)
  line L612 (-4.2174, -4.9877) -> (-3.5343, -4.4918)
  line L613 (-3.5343, -4.4918) -> (-2.8928, -3.8671)
  line L614 (-2.8928, -3.8671) -> (-2.8791, -3.071)
  line L615 (-2.8791, -3.071) -> (-3.0412, -2.3552)
  line L616 (-3.0412, -2.3552) -> (-3.2475, -2.2788)
  line L617 (-3.2475, -2.2788) -> (-3.6314, -2.2928)
  line L618 (-3.6314, -2.2928) -> (-4.2387, -2.3633)
  line L619 (-4.2387, -2.3633) -> (-4.5212, -2.5772)
  line L620 (-4.5212, -2.5772) -> (-4.7219, -2.9016)
  line L621 (-4.7219, -2.9016) -> (-4.757, -3.7452)
  line L622 (-4.757, -3.7452) -> (-4.7333, -4.5849)
  line L623 (-4.7333, -4.5849) -> (-4.5225, -4.8817)
  line L624 (11.5347, -4.7676) -> (12.27, -5.3998)
  line L625 (12.27, -5.3998) -> (12.6476, -5.512)
  line L626 (12.6476, -5.512) -> (12.7867, -5.0157)
  line L627 (12.7867, -5.0157) -> (12.8065, -3.8221)
  line L628 (12.8065, -3.8221) -> (12.7697, -1.9988)
  line L629 (12.7697, -1.9988) -> (12.6827, -1.7942)
  line L630 (12.6827, -1.7942) -> (12.5132, -1.8094)
  line L631 (12.5132, -1.8094) -> (12.1343, -1.9898)
  line L632 (12.1343, -1.9898) -> (11.2414, -2.7549)
  line L633 (11.2414, -2.7549) -> (10.6955, -3.2716)
  line L634 (10.6955, -3.2716) -> (10.5441, -3.6535)
  line L635 (10.5441, -3.6535) -> (10.8146, -4.0893)
  line L636 (10.8146, -4.0893) -> (11.5347, -4.7676)
  line L637 (3.0035, -4.0457) -> (3.1605, -4.6314)
  line L638 (3.1605, -4.6314) -> (3.3527, -4.8376)
  line L639 (3.3527, -4.8376) -> (3.7058, -4.6743)
  line L640 (3.7058, -4.6743) -> (4.3457, -4.1513)
  line L641 (4.3457, -4.1513) -> (5.2947, -3.3229)
  line L642 (5.2947, -3.3229) -> (5.3822, -3.1913)
  line L643 (5.3822, -3.1913) -> (5.3355, -3.1191)
  line L644 (5.3355, -3.1191) -> (4.286, -2.831)
  line L645 (4.286, -2.831) -> (3.4279, -2.6889)
  line L646 (3.4279, -2.6889) -> (3.0544, -2.8251)
  line L647 (3.0544, -2.8251) -> (2.8889, -2.9468)
  line L648 (2.8889, -2.9468) -> (2.8285, -3.1145)
  line L649 (2.8285, -3.1145) -> (3.0035, -4.0457)
  line L650 (1.213, -5.1681) -> (1.2832, -6.0508)
  line L651 (1.2832, -6.0508) -> (1.5228, -6.699)
  line L652 (1.5228, -6.699) -> (1.8062, -7.2319)
  line L653 (1.8062, -7.2319) -> (2.1825, -7.308)
  line L654 (2.1825, -7.308) -> (2.4139, -7.291)
  line L655 (2.4139, -7.291) -> (2.5646, -7.1719)
  line L656 (2.5646, -7.1719) -> (2.8886, -6.2192)
  line L657 (2.8886, -6.2192) -> (3.1329, -5.1344)
  line L658 (3.1329, -5.1344) -> (2.9569, -4.0741)
  line L659 (2.9569, -4.0741) -> (2.7176, -3.1454)
  line L660 (2.7176, -3.1454) -> (2.5194, -2.9823)
  line L661 (2.5194, -2.9823) -> (2.2797, -3.0325)
  line L662 (2.2797, -3.0325) -> (1.7496, -3.5965)
  line L663 (1.7496, -3.5965) -> (1.2486, -4.2802)
  line L664 (1.2486, -4.2802) -> (1.213, -5.1681)
  line L665 (0.1066, -5.1281) -> (1.0588, -5.8127)
  line L666 (1.0588, -5.8127) -> (1.1664, -5.6464)
  line L667 (1.1664, -5.6464) -> (1.16, -5.1429)
  line L668 (1.16, -5.1429) -> (1.0753, -4.3051)
  line L669 (1.0753, -4.3051) -> (0.7272, -3.814)
  line L670 (0.7272, -3.814) -> (0.3184, -3.4522)
  line L671 (0.3184, -3.4522) -> (-0.1916, -3.5201)
  line L672 (-0.1916, -3.5201) -> (-0.6694, -3.677)
  line L673 (-0.6694, -3.677) -> (-0.853, -3.9386)
  line L674 (-0.853, -3.9386) -> (-0.9137, -4.1142)
  line L675 (-0.9137, -4.1142) -> (-0.834, -4.2966)
  line L676 (-0.834, -4.2966) -> (0.1066, -5.1281)
  line L677 (5.9755, -5.1295) -> (6.2406, -6.1952)
  line L678 (6.2406, -6.1952) -> (6.4544, -6.5774)
  line L679 (6.4544, -6.5774) -> (6.7298, -6.3005)
  line L680 (6.7298, -6.3005) -> (7.1796, -5.3887)
  line L681 (7.1796, -5.3887) -> (7.839, -3.9424)
  line L682 (7.839, -3.9424) -> (7.857, -3.5867)
  line L683 (7.857, -3.5867) -> (7.683, -3.4069)
  line L684 (7.683, -3.4069) -> (6.9977, -3.1918)
  line L685 (6.9977, -3.1918) -> (6.2803, -3.0155)
  line L686 (6.2803, -3.0155) -> (5.8823, -3.1065)
  line L687 (5.8823, -3.1065) -> (5.6899, -3.2144)
  line L688 (5.6899, -3.2144) -> (5.6354, -3.4611)
  line L689 (5.6354, -3.4611) -> (5.9755, -5.1295)
  line L690 (-8.3627, -4.2464) -> (-8.1266, -4.7379)
  line L691 (-8.1266, -4.7379) -> (-7.6061, -5.1709)
  line L692 (-7.6061, -5.1709) -> (-7.0472, -5.4786)
  line L693 (-7.0472, -5.4786) -> (-6.5428, -5.0925)
  line L694 (-6.5428, -5.0925) -> (-6.1471, -4.5906)
  line L695 (-6.1471, -4.5906) -> (-6.3489, -4.0873)
  line L696 (-6.3489, -4.0873) -> (-6.538, -3.7974)
  line L697 (-6.538, -3.7974) -> (-6.7315, -3.6567)
  line L698 (-6.7315, -3.6567) -> (-7.6008, -3.6644)
  line L699 (-7.6008, -3.6644) -> (-8.4089, -3.7977)
  line L700 (-8.4089, -3.7977) -> (-8.4569, -3.9553)
  line L701 (-8.4569, -3.9553) -> (-8.3627, -4.2464)
  line L702 (9.3715, -5.8467) -> (9.4772, -6.6916)
  line L703 (9.4772, -6.6916) -> (9.6986, -7.1254)
  line L704 (9.6986, -7.1254) -> (10.2031, -7.2852)
  line L705 (10.2031, -7.2852) -> (11.1584, -7.3081)
  line L706 (11.1584, -7.3081) -> (12.6008, -7.2257)
  line L707 (12.6008, -7.2257) -> (12.7812, -7.0297)
  line L708 (12.7812, -7.0297) -> (12.8069, -6.6481)
  line L709 (12.8069, -6.6481) -> (12.7867, -6.2481)
  line L710 (12.7867, -6.2481) -> (12.6449, -5.9239)
  line L711 (12.6449, -5.9239) -> (11.5104, -4.8154)
  line L712 (11.5104, -4.8154) -> (10.2543, -3.8326)
  line L713 (10.2543, -3.8326) -> (9.9699, -3.8148)
  line L714 (9.9699, -3.8148) -> (9.6864, -4.0122)
  line L715 (9.6864, -4.0122) -> (9.4265, -4.2508)
  line L716 (9.4265, -4.2508) -> (9.3071, -4.5214)
  line L717 (9.3071, -4.5214) -> (9.3715, -5.8467)
  line L718 (6.3762, -7.2028) -> (5.9328, -5.1749)
  line L719 (5.9328, -5.1749) -> (5.6573, -4.0781)
  line L720 (5.6573, -4.0781) -> (5.4026, -3.6108)
  line L721 (5.4026, -3.6108) -> (5.0222, -3.6816)
  line L722 (5.0222, -3.6816) -> (4.3694, -4.1989)
  line L723 (4.3694, -4.1989) -> (3.353, -5.1626)
  line L724 (3.353, -5.1626) -> (2.9403, -6.2269)
  line L725 (2.9403, -6.2269) -> (2.7891, -6.8519)
  line L726 (2.7891, -6.8519) -> (2.9012, -7.1729)
  line L727 (2.9012, -7.1729) -> (3.423, -7.2911)
  line L728 (3.423, -7.2911) -> (4.5006, -7.308)
  line L729 (4.5006, -7.308) -> (6.1394, -7.2949)
  line L730 (6.1394, -7.2949) -> (6.3762, -7.2028)
  line L731 (9.319, -5.8493) -> (9.1236, -4.5358)
  line L732 (9.1236, -4.5358) -> (8.9312, -4.2878)
  line L733 (8.9312, -4.2878) -> (8.5837, -4.0928)
  line L734 (8.5837, -4.0928) -> (8.2262, -3.9464)
  line L735 (8.2262, -3.9464) -> (7.9638, -4.0388)
  line L736 (7.9638, -4.0388) -> (7.2086, -5.4483)
  line L737 (7.2086, -5.4483) -> (6.7794, -6.5235)
  line L738 (6.7794, -6.5235) -> (6.7125, -7.0756)
  line L739 (6.7125, -7.0756) -> (7.077, -7.279)
  line L740 (7.077, -7.279) -> (7.9414, -7.3081)
  line L741 (7.9414, -7.3081) -> (8.8159, -7.2854)
  line L742 (8.8159, -7.2854) -> (9.251, -7.1259)
  line L743 (9.251, -7.1259) -> (9.3759, -6.6929)
  line L744 (9.3759, -6.6929) -> (9.319, -5.8493)
  line L745 (-4.0439, -6.22) -> (-3.9096, -6.849)
  line L746 (-3.9096, -6.849) -> (-3.7517, -7.172)
  line L747 (-3.7517, -7.172) -> (-3.4684, -7.291)
  line L748 (-3.4684, -7.291) -> (-2.9579, -7.308)
  line L749 (-2.9579, -7.308) -> (-2.4473, -7.286)
  line L750 (-2.4473, -7.286) -> (-2.1633, -7.1316)
  line L751 (-2.1633, -7.1316) -> (-2.0038, -6.7125)
  line L752 (-2.0038, -6.7125) -> (-1.8663, -5.8964)
  line L753 (-1.8663, -5.8964) -> (-1.748, -4.627)
  line L754 (-1.748, -4.627) -> (-1.8887, -4.3914)
  line L755 (-1.8887, -4.3914) -> (-2.2049, -4.2112)
  line L756 (-2.2049, -4.2112) -> (-2.5361, -4.0623)
  line L757 (-2.5361, -4.0623) -> (-2.782, -4.0464)
  line L758 (-2.782, -4.0464) -> (-3.5051, -4.5348)
  line L759 (-3.5051, -4.5348) -> (-3.934, -4.8971)
  line L760 (-3.934, -4.8971) -> (-4.133, -5.1934)
  line L761 (-4.133, -5.1934) -> (-4.1529, -5.5817)
  line L762 (-4.1529, -5.5817) -> (-4.0439, -6.22)
  line L763 (1.471, -6.71) -> (1.1013, -6.0707)
  line L764 (1.1013, -6.0707) -> (0.0918, -5.1833)
  line L765 (0.0918, -5.1833) -> (-0.9208, -4.3853)
  line L766 (-0.9208, -4.3853) -> (-1.1284, -4.3184)
  line L767 (-1.1284, -4.3184) -> (-1.3123, -4.3715)
  line L768 (-1.3123, -4.3715) -> (-1.4822, -4.4611)
  line L769 (-1.4822, -4.4611) -> (-1.591, -4.65)
  line L770 (-1.591, -4.65) -> (-1.8142, -5.8982)
  line L771 (-1.8142, -5.8982) -> (-1.9084, -6.7133)
  line L772 (-1.9084, -6.7133) -> (-1.7661, -7.1318)
  line L773 (-1.7661, -7.1318) -> (-1.2311, -7.286)
  line L774 (-1.2311, -7.286) -> (-0.147, -7.308)
  line L775 (-0.147, -7.308) -> (1.466, -7.2333)
  line L776 (1.466, -7.2333) -> (1.5936, -7.0558)
  line L777 (1.5936, -7.0558) -> (1.471, -6.71)
  point P0 (2.1873, -19.4723)
  constraints: 1556 end point, 17 parallel, 17 perpendicular
body "Solid1"
